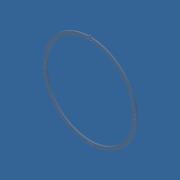
# Autodesk Inventor part: J005536
Saved by Autodesk Inventor 2018.2 (Build 222227000, 227)
## iProperties
Created: 2014-10-13
Material: ACRYLIC, CLEAR
Vendor: HHMI: JFRC - ID&F
Document SubType Name: Modeling
Designer: negrashovi
Mass: 1.91647 g
Surface Area: 42.4442 cm^2
Volume: 2.90374 cm^3
Density: 0.66 g/cm^3
Project: P-75301
Part Number: J005536
Description: RING FOR ROUND INSERT
Appearance: Polycarbonate - Clear
RuleStatus: InUse
AfterDocSave0: file://Part Number Cleaner
LAB/DEPT: RUBIN (LAB)
REQUESTING SCIENTIST: ASO, YOSHI
SURFACE ROUGHNESS: N/A
DESIGN DEPARTMENT: HHMI: JRC - ID&F
SPECIAL FINISH: NONE
ALTERED ITEM PART NUMBER: N/A
ALTERED ITEM VENDOR: N/A
ALTERED ITEM DESCRIPTION: N/A
Author: negrashovi
Revision Number: B
Autodesk Inventor part; units mm, degrees
ref_plane "YZ Plane" through (0, 0, 0) normal (1, 0, 0) x (0, 1, 0)
ref_plane "XZ Plane" through (0, 0, 0) normal (0, 1, 0) x (-1, 0, 0)
ref_plane "XY Plane" through (0, 0, 0) normal (0, 0, 1) x (1, 0, 0)
sketch "Sketch1" plane through (0, 0, 0) normal (0, 0, 1) x (1, 0, 0)
  arc A0 (-1.5875, 55.2682) -> (1.5875, 55.2682) centre (0, 0) ccw
  circle A1 centre (0, 0) radius 50.8
  line L0 (0, 79.3124) -> (0, -77.7249) construction
  line L1 (-77.4074, 0) -> (77.4074, 0) construction
  circle A2 centre (0, 0) radius 52.8955 construction
  circle A3 centre (-1.846, 52.8633) radius 0.75
  circle A4 centre (1.846, 52.8633) radius 0.75
  circle A5 centre (-52.8633, -1.846) radius 0.75
  circle A6 centre (-52.8633, 1.846) radius 0.75
  circle A7 centre (1.846, -52.8633) radius 0.75
  circle A8 centre (-1.846, -52.8633) radius 0.75
  circle A9 centre (52.8633, 1.846) radius 0.75
  circle A10 centre (52.8633, -1.846) radius 0.75
  arc A11 (1.5875, 55.291) -> (-1.5875, 55.291) centre (0, 55.291) ccw
  line L2 (-1.5875, 55.291) -> (-1.5875, 55.2682)
  line L3 (1.5875, 55.291) -> (1.5875, 55.2682)
  dimension "d0" = 110.582
  dimension "d1" = 101.6
  dimension "d4" = 105.791
  dimension "d5" = 4
  dimension "d6" = 1.5
  dimension "d9" = 360
  dimension "d11" = 3.175
  constraints: 12 centre point, 7 point on circle, 4 end point, 3 coincident, 2 tangent, 1 parallel, 1 perpendicular, 1 point on line, 18 other
  measures "d0" diameter of A0
  measures "d1" diameter of A1
  measures "d4" diameter of A2
  measures "d6" diameter of A4
  measures "d11" diameter of A11
extrude "Extrusion1" add sketch "Sketch1" against normal blind 1.5
body "Solid1"
